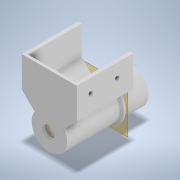
# Autodesk Inventor part: CTF_GOOT
Saved by Autodesk Inventor 2020.5 (Build 245400000, 400)
## iProperties
Created: 2022-03-21
Part Number: CTF_GOOT
Material: Generic
Document SubType Name: Modeling
Designer: EDDY
Density: 1 g/cm^3
Appearance: Default
Author: EDDY
Autodesk Inventor part; units mm, degrees
ref_plane "YZ Plane" through (0, 0, 0) normal (1, 0, 0) x (0, 1, 0)
ref_plane "XZ Plane" through (0, 0, 0) normal (0, 1, 0) x (-1, 0, 0)
ref_plane "XY Plane" through (0, 0, 0) normal (0, 0, 1) x (1, 0, 0)
ref_plane "Work Plane1" through (0, 0, 0) normal (0, 0, 1) x (1, 0, 0)
sketch "Sketch1" plane through (0, 0, 0) normal (0, 0, 1) x (1, 0, 0)
  circle A0 centre (0, -20.2) radius 20.2 construction
  circle A1 centre (0, -20.2) radius 17.5 construction
  circle A2 centre (0, -20.2) radius 17
  circle A3 centre (0, -20.2) radius 20
  line L0 (0, -8.211) -> (0, -3.7)
  point P0 (0, 0)
  point P1 (0, -3.2)
  dimension "d2" = 34
  dimension "d0" = 40
  dimension "d3" = 16.5
  constraints: 2 coincident, 2 end point, 2 vertical alignment, 1 centre point, 2 other
  measures "d0" diameter of A3
  measures "d3" distance of L0.end point (0, -20.2)
extrude "Extrusion1" add sketch "Sketch1" against normal blind 28
sketch "Sketch2" plane through (0, -20.2, 0) normal (0, 0, 1) x (1, 0, 0)
  line L0 (0, 0) -> (-54.4536, 54.4536) construction
  line L1 (0, 0) -> (55.7945, 55.7945) construction
  line L2 (0, 11.989) -> (0, 16.5) construction
  circle A0 centre (0, 0) radius 17 projected
  line L3 (-12.0208, 12.0208) -> (-14.1421, 14.1421)
  circle A1 centre (0, 0) radius 20 projected
  line L4 (14.1421, 14.1421) -> (12.0208, 12.0208)
  line L5 (31, 60) -> (31, 25.3431)
  line L6 (31, 25.3431) -> (16.6848, 11.028)
  line L7 (31, 60) -> (27, 60)
  line L8 (12.0208, 12.0208) -> (27, 27)
  line L9 (27, 27) -> (27, 60)
  line L10 (0, 11.989) -> (0, 16.5)
  line L11 (0, 11.989) -> (0, 16.5)
  line L12 (0, 0) -> (0, 35.2137) construction
  line L13 (-31, 60) -> (-31, 25.3431)
  line L14 (-31, 25.3431) -> (-16.6848, 11.028)
  line L15 (-31, 60) -> (-27, 60)
  line L16 (-12.0208, 12.0208) -> (-27, 27)
  line L17 (-27, 27) -> (-27, 60)
  point P0 (0, 20.2)
  point P1 (-14.1421, 14.1421)
  dimension "d6" = 90
  dimension "d7" = 45
  dimension "d12" = 4
  dimension "d13" = 4
  dimension "d15" = 60
  constraints: 34 end point, 7 point on line, 6 symmetric about line, 5 point on circle, 3 vertical, 1 horizontal, 1 parallel, 1 perpendicular, 2 other
  measures "d6" angle of L1 L0
  measures "d7" angle of L0 L2
  measures "d12" distance between parallel lines of L1 L6
  measures "d13" distance of L5.start L7.end
  measures "d15" distance from line of L7 A0.centre
ref_plane "Work Plane2" through (-10, -30.2, 60) normal (0, 0, 1) x (1, 0, 0)
ref_plane "Work Plane3" through (0, -30.2, 60.5) normal (0, 0, 1) x (0, 1, 0)
extrude "Extrusion2" add sketch "Sketch2" along normal up to surface (60.5 mm away) contours A0 L4 A1 L3 | L8 L9 L7 L5 L6 A1 | A1 L14 L13 L15 L17 L16 picked at (18.6256, -3.0158)
fillet "Fillet1" radius 2 1 edges at (-12.0208, -8.1792, 30.25)
fillet "Fillet2" radius 2 1 edges at (12.0208, -8.1792, 30.25)
sketch "Sketch4" plane through (0, -20.2, 60.5) normal (0, 0, 1) x (1, 0, 0)
  line L0 (-27, 60) -> (-31, 60) projected
  line L1 (-31, 60) -> (31, 60)
  line L2 (-31, 25.3431) -> (-31, 60) projected
  line L3 (-16.6848, 11.028) -> (-31, 25.3431) projected
  arc A0 (-16.6848, 11.028) -> (16.6848, 11.028) centre (0, 0) ccw projected
  line L4 (31, 25.3431) -> (16.6848, 11.028) projected
  line L5 (31, 60) -> (31, 25.3431) projected
  circle A1 centre (0, 0) radius 6 projected
  circle A2 centre (0, 0) radius 4.1871
  point P0 (0, 20.2)
  point P1 (-27, 60)
  constraints: 2 end point, 1 centre point, 1 coincident, 1 horizontal
extrude "Extrusion3" add sketch "Sketch4" along normal blind 3 contours L1 L5 L4 A0 L3 L2 L0
thicken "Thicken1" operation add thickness 0.25 both sides no extend neighbours yes toward (0.9967573, -0.0804666, 0) faces at (5.9805, -20.6828, 62.5)
sketch "Sketch5" plane through (27, 6.8, 0) normal (-1, 0, 0) x (0, 0, 1)
  line L0 (0, 33) -> (60.5, 33) projected
  line L1 (63.5, -1.6569) -> (63.5, 33) projected
  circle A0 centre (18.5, 18) radius 2
  circle A1 centre (48.5, 18) radius 2
  point P0 (0, -6.8)
  dimension "d22" = 15
  dimension "d23" = 15
  dimension "d24" = 30
  dimension "d25" = 4
  dimension "d26" = 4
  constraints: 3 coincident, 2 centre point
  measures "d22" distance from line of L0 point (48.5, 18)
  measures "d23" distance from line of point (48.5, 18) L1
  measures "d24" distance of point (18.5, 18) point (48.5, 18)
  measures "d25" diameter of A0
  measures "d26" diameter of A1
extrude "Extrusion4" cut sketch "Sketch5" against normal blind 10
ref_plane "Work Plane4" through (0, 0, 0) normal (0, 0, 1) x (1, 0, 0)
sketch "Sketch6" plane through (0, 0, 0) normal (0, 0, 1) x (1, 0, 0)
  line L0 (-31, 5.1431) -> (-16.6848, -9.172) projected
  circle A0 centre (0, -20.2) radius 22.6 projected
  arc A1 (-16.6848, -9.172) -> (16.6848, -9.172) centre (0, -20.2) ccw projected
  line L1 (-16.6848, -9.172) -> (-18.5567, -7.3001)
  line L2 (16.6848, -9.172) -> (31, 5.1431) projected
  line L3 (18.5567, -7.3001) -> (16.6848, -9.172)
  point P0 (0, 0)
  constraints: 4 end point, 2 point on circle, 2 point on line, 1 collinear
extrude "Extrusion5" add sketch "Sketch6" along normal blind 4 contours L0 A1 L2 A0 picked at (-21.5536, -21.3519)
chamfer "Chamfer1" distance 2 angle 45 1 edges at (0, -42.8, 4)
fillet "Fillet3" radius 2 1 edges at (0, -40.2, 4)
equation "\"d7\" = 0.5 * d6"
body "Solid1"
